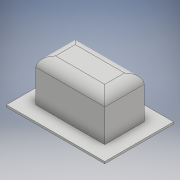
# Autodesk Inventor part: powerbutton
Saved by Autodesk Inventor 2017 SP1 (Build 210196100, 196)
## iProperties
Created: 2017-10-10
Part Number: powerbutton
Material: Generic
Document SubType Name: Modeling
Designer: Groguard
Density: 1 g/cm^3
Appearance: Default
Author: Groguard
Autodesk Inventor part; units mm, degrees
ref_plane "YZ Plane" through (0, 0, 0) normal (1, 0, 0) x (0, 1, 0)
ref_plane "XZ Plane" through (0, 0, 0) normal (0, 1, 0) x (-1, 0, 0)
ref_plane "XY Plane" through (0, 0, 0) normal (0, 0, 1) x (1, 0, 0)
sketch "Sketch1" plane through (0, 0, 0) normal (0, 0, 1) x (1, 0, 0)
  line L0 (-1, 6) -> (9, 6)
  line L1 (9, 6) -> (9, -1)
  line L2 (9, -1) -> (-1, -1)
  line L3 (-1, -1) -> (-1, 6)
  line L4 (0.5, 4.5) -> (7.5, 4.5)
  line L5 (7.5, 4.5) -> (7.5, 0.5)
  line L6 (7.5, 0.5) -> (0.5, 0.5)
  line L7 (0.5, 0.5) -> (0.5, 4.5)
  point P0 (0, 0)
  constraints: 16 end point, 4 parallel, 2 perpendicular
extrude "Extrusion1" add sketch "Sketch1" along normal blind 4.5 contours L0 L1 L2 L3 | L4 L5 L6 L7
sketch "Sketch2" plane through (0, 0, 4.5) normal (0, 0, 1) x (1, 0, 0)
  line L0 (-1, 6) -> (9, 6)
  line L1 (9, 6) -> (9, -1)
  line L2 (9, -1) -> (-1, -1)
  line L3 (-1, -1) -> (-1, 6)
  line L4 (0.5, 4.5) -> (7.5, 4.5)
  line L5 (7.5, 4.5) -> (7.5, 0.5)
  line L6 (7.5, 0.5) -> (0.5, 0.5)
  line L7 (0.5, 0.5) -> (0.5, 4.5)
  point P0 (0, 0)
  point P1 (0, 0)
  constraints: 16 end point, 4 parallel, 2 perpendicular
extrude "Extrusion2" cut sketch "Sketch2" against normal blind 4.3
fillet "Fillet1" radius 1 4 edges at (0.5, 2.5, 4.5) (4, 0.5, 4.5) (7.5, 2.5, 4.5) (4, 4.5, 4.5)
body "Solid1"
